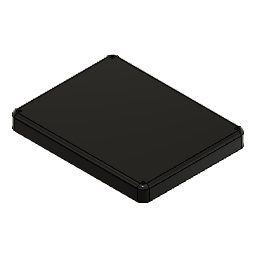
electronic_box (Autodesk Fusion 360 design; units mm, degrees)
Autodesk Fusion 360 part; units mm, degrees
note: some values were not read from the file. Set by a fixed rule: which sketch regions a step uses; which face or edge a step refers to.
sketch "Esquisse1" plane through (0, 0, 0) normal (0, 1, 0) x (1, 0, 0)
  line L0 (-100, 85) -> (100, 85)
  line L1 (110, 75) -> (110, -75)
  line L2 (100, -85) -> (-100, -85)
  line L3 (-110, -75) -> (-110, 75)
  line L4 (-110, 85) -> (110, -85) construction
  line L5 (110, 85) -> (-110, -85) construction
  arc A0 (-100, 85) -> (-110, 75) centre (-100, 75) ccw
  arc A1 (110, 75) -> (100, 85) centre (100, 75) ccw
  arc A2 (100, -85) -> (110, -75) centre (100, -75) ccw
  arc A3 (-110, -75) -> (-100, -85) centre (-100, -75) ccw
  arc A4 (-100, 82) -> (-107, 75) centre (-100, 75) ccw
  line L6 (-107, -75) -> (-107, 75)
  arc A5 (-107, -75) -> (-100, -82) centre (-100, -75) ccw
  line L7 (100, -82) -> (-100, -82)
  arc A6 (100, -82) -> (107, -75) centre (100, -75) ccw
  line L8 (107, 75) -> (107, -75)
  arc A7 (107, 75) -> (100, 82) centre (100, 75) ccw
  line L9 (-100, 82) -> (100, 82)
  dimension "d8" = 170
  dimension "d9" = 220
  dimension "d10" = 10
  dimension "d11" = 3
  constraint horizontal L0
  constraint perpendicular L0 L1
  constraint parallel L0 L2
  constraint parallel L1 L3
  constraint coincident L4 origin
  constraint coincident L5 origin
  constraint coincident L4.start L3
  constraint coincident L4.start L0
  constraint tangent L3 A0
  constraint tangent L0 A0
  constraint coincident L5.start L0
  constraint coincident L5.start L1
  constraint tangent L0 A1
  constraint tangent L1 A1
  constraint equal A0 A1
  constraint coincident L4.end L2
  constraint coincident L4.end L1
  constraint tangent L2 A2
  constraint tangent L1 A2
  constraint equal A0 A2
  constraint coincident L5.end L2
  constraint coincident L5.end L3
  constraint tangent L2 A3
  constraint tangent L3 A3
  constraint equal A0 A3
  measures "d8" distance of L4.start L5.end
  measures "d9" distance of L4.end L5.end
  measures "d10" radius of A0
extrude "Extrusion2" add sketch "Esquisse1" along normal blind 20 makes body 1
sketch "Esquisse2" plane through (0, 20, 0) normal (0, 1, 0) x (-1, 0, 0)
  arc A0 (107, 75) -> (100, 82) centre (100, 75) ccw
  line L0 (107, 75) -> (107, -75)
  arc A1 (100, -82) -> (107, -75) centre (100, -75) ccw
  line L1 (100, -82) -> (-100, -82)
  arc A2 (-107, -75) -> (-100, -82) centre (-100, -75) ccw
  line L2 (-107, -75) -> (-107, 75)
  arc A3 (-100, 82) -> (-107, 75) centre (-100, 75) ccw
  line L3 (-100, 82) -> (100, 82)
  arc A4 (100, -85) -> (110, -75) centre (100, -75) ccw
  line L4 (110, -75) -> (110, 75)
  arc A5 (110, 75) -> (100, 85) centre (100, 75) ccw
  line L5 (100, 85) -> (-100, 85)
  arc A6 (-100, 85) -> (-110, 75) centre (-100, 75) ccw
  line L6 (-110, 75) -> (-110, -75)
  arc A7 (-110, -75) -> (-100, -85) centre (-100, -75) ccw
  line L7 (-100, -85) -> (100, -85)
  line L8 (-110, 75) -> (-110, -75)
  arc A8 (-100, 85) -> (-110, 75) centre (-100, 75) ccw
  line L9 (100, 85) -> (-100, 85)
  circle A9 centre (100, 75) radius 0.001
  line L10 (110, -75) -> (110, 75)
  arc A10 (100, -85) -> (110, -75) centre (100, -75) ccw
  line L11 (-100, -85) -> (100, -85)
  circle A11 centre (-100, -75) radius 0.001
extrude "Extrusion3" add sketch "Esquisse2" along normal blind 3 contours A0 L0 A1 L1 A2 L2 A3 L3 | A4 L4 A5 L5 A6 L6 A7 L7 L8 A8 L9 L10 A10 L11 | A9 | A11 bodies 1
fillet "Congé1" radius 2 8 edges at (0, 20, -82) (104.9497, 20, -79.9497) (107, 20, 0) (104.9497, 20, 79.9497) (0, 20, 82) (-104.9497, 20, 79.9497) (-107, 20, 0) (-104.9497, 20, -79.9497) on bodies 1
fillet "Congé2" radius 5 8 edges at (0, 23, 85) (107.0711, 23, 82.0711) (110, 23, 0) (107.0711, 23, -82.0711) (0, 23, -85) (-107.0711, 23, -82.0711) (-110, 23, 0) (-107.0711, 23, 82.0711) on bodies 1
sketch "Esquisse3" plane through (0, 0, -85) normal (0, 0, -1) x (-1, 0, 0)
  line L0 (100, 18) -> (-100, 18)
  line L1 (-100, 18) -> (-100, 0)
  line L2 (-100, 0) -> (100, 0)
  line L3 (100, 0) -> (100, 18)
  line L4 (-58.4785, 6.134) -> (-73.4785, 6.134)
  line L5 (-73.4785, 6.134) -> (-73.4785, 13.134)
  line L6 (-73.4785, 13.134) -> (-58.4785, 13.134)
  line L7 (-58.4785, 13.134) -> (-58.4785, 6.134)
  line L8 (-39.7725, 5.6821) -> (-51.7725, 5.6821)
  line L9 (-51.7725, 5.6821) -> (-51.7725, 13.6821)
  line L10 (-51.7725, 13.6821) -> (-39.7725, 13.6821)
  line L11 (-39.7725, 13.6821) -> (-39.7725, 5.6821)
  circle A0 centre (-32.676, 9.0787) radius 2.5
  dimension "d20" = 15
  dimension "d21" = 7
  dimension "d24" = 12
  dimension "d25" = 8
  dimension "d26" = 5
  constraint horizontal L4
  constraint vertical L5
  constraint horizontal L6
  constraint vertical L7
  constraint horizontal L8
  constraint vertical L9
  constraint horizontal L10
  constraint vertical L11
  measures "d20" distance of L4.start L4.end
  measures "d21" distance of L4.start L6.end
  measures "d24" distance of L8.start L8.end
  measures "d25" distance of L8.start L10.end
  measures "d26" diameter of A0
extrude "Extrusion4" cut sketch "Esquisse3" against normal blind 30 contours L4 L5 L6 L7 | L8 L9 L10 L11 | A0 bodies 1
sketch "Esquisse4" plane through (0, 0, 0) normal (0, -1, 0) x (1, 0, 0)
  arc A0 (-100, 82) -> (-107, 75) centre (-100, 75) ccw
  line L0 (-100, 82) -> (100, 82)
  arc A1 (107, 75) -> (100, 82) centre (100, 75) ccw
  line L1 (107, 75) -> (107, -75)
  arc A2 (100, -82) -> (107, -75) centre (100, -75) ccw
  line L2 (100, -82) -> (-100, -82)
  arc A3 (-107, -75) -> (-100, -82) centre (-100, -75) ccw
  line L3 (-107, -75) -> (-107, 75)
  arc A4 (-110, -75) -> (-100, -85) centre (-100, -75) ccw
  line L4 (-100, -85) -> (100, -85)
  arc A5 (100, -85) -> (110, -75) centre (100, -75) ccw
  line L5 (110, -75) -> (110, 75)
  arc A6 (110, 75) -> (100, 85) centre (100, 75) ccw
  line L6 (100, 85) -> (-100, 85)
  arc A7 (-100, 85) -> (-110, 75) centre (-100, 75) ccw
  line L7 (-110, 75) -> (-110, -75)
sketch "Esquisse5" plane through (0, 20, 0) normal (0, -1, 0) x (1, 0, 0)
  line L0 (-100, -80) -> (100, -80)
  line L1 (105, -75) -> (105, 75)
  line L2 (100, 80) -> (-100, 80)
  line L3 (-105, 75) -> (-105, -75)
  circle A0 centre (-101, 76) radius 2
  circle A1 centre (-101, 76) radius 2
  circle A2 centre (-101, 76) radius 3
  line L4 (0, 100) -> (0, -84.8494) construction
  line L5 (-132.4366, 0.0945) -> (95, 0.0945) construction
  circle A3 centre (101, 76) radius 3
  circle A4 centre (101, 76) radius 2
  circle A5 centre (101, -75.811) radius 3
  circle A6 centre (101, -75.811) radius 2
  circle A7 centre (-101, -75.811) radius 3
  circle A8 centre (-101, -75.811) radius 2
  arc A9 (100, -80) -> (105, -75) centre (100, -75) ccw
  arc A10 (105, 75) -> (100, 80) centre (100, 75) ccw
  arc A11 (-100, 80) -> (-105, 75) centre (-100, 75) ccw
  arc A12 (-105, -75) -> (-100, -80) centre (-100, -75) ccw
  point P0 (-101, -75.811)
  dimension "d27" = 4
  dimension "d28" = 4
  dimension "d29" = 6
  dimension "d30" = 4
  dimension "d31" = 4
  dimension "d32" = 4
  dimension "d33" = 4
  constraint concentric A0 A2
  constraint perpendicular L2 L4
  constraint perpendicular L1 L5
  constraint symmetric A0 L4 A4
  constraint symmetric A2 L4 A3
  constraint symmetric A0 L5 A8
  constraint symmetric A0.centre L5 P0
  constraint symmetric A2 L5 A7
  constraint symmetric L5 A3 A5
  constraint symmetric L5 A4 A6
  measures "d27" diameter of A0
  measures "d28" diameter of A1
  measures "d29" diameter of A2
  measures "d30" distance of L2 A0.centre
  measures "d31" distance of L2 A0.centre
  measures "d32" distance of L3 A0.centre
  measures "d33" distance of L3 A0.centre
extrude "Extrusion5" add sketch "Esquisse5" along normal up to surface (20 mm away) contours A2 | A3 | A5 | A7 bodies 1
extrude "Extrusion6" cut sketch "Esquisse5" against normal blind 55 contours A0 A1 | A4 | A6 | A8 bodies 1
sketch "Esquisse6" plane through (0, 0, -85) normal (0, 0, -1) x (-1, 0, 0)
  line L0 (-73.4785, 6.134) -> (-73.4785, 13.134)
  line L1 (-73.4785, 13.134) -> (-58.4785, 13.134)
  line L2 (-58.4785, 13.134) -> (-58.4785, 6.134)
  line L3 (-58.4785, 6.134) -> (-73.4785, 6.134)
  line L4 (-51.7725, 5.6821) -> (-51.7725, 13.6821)
  line L5 (-51.7725, 13.6821) -> (-39.7725, 13.6821)
  line L6 (-39.7725, 13.6821) -> (-39.7725, 5.6821)
  line L7 (-39.7725, 5.6821) -> (-51.7725, 5.6821)
  circle A0 centre (-32.676, 9.0787) radius 2.5
  line L8 (100, 18) -> (-100, 18)
  line L9 (-100, 18) -> (-100, 0)
  line L10 (-100, 0) -> (100, 0)
  line L11 (100, 0) -> (100, 18)
  line L12 (95, 0) -> (10, 0)
  line L13 (10, 0) -> (10, 18)
  line L14 (10, 18) -> (95, 18)
  line L15 (95, 18) -> (95, 0)
  dimension "d39" = 85
  dimension "d45" = 5
  constraint horizontal L12
  constraint vertical L13
  constraint horizontal L14
  constraint vertical L15
  constraint coincident L8 L13.end
  constraint coincident L10 L12.start
  measures "d39" distance of L13 L15
  measures "d45" distance of L11 L15
extrude "Extrusion7" cut sketch "Esquisse6" against normal blind 25 contours L8 L10 L12 L13 L14 L15 bodies 1
sketch "Esquisse7" plane through (0, 0, 0) normal (0, -1, 0) x (1, 0, 0)
  line L0 (-95, -85) -> (-95, -82)
  line L1 (-95, -82) -> (-100, -82)
  arc A0 (-107, -75) -> (-100, -82) centre (-100, -75) ccw
  line L2 (-107, -75) -> (-107, 75)
  arc A1 (-100, 82) -> (-107, 75) centre (-100, 75) ccw
  line L3 (-100, 82) -> (100, 82)
  arc A2 (107, 75) -> (100, 82) centre (100, 75) ccw
  line L4 (107, 75) -> (107, -75)
  arc A3 (100, -82) -> (107, -75) centre (100, -75) ccw
  line L5 (100, -82) -> (-10, -82)
  line L6 (-10, -82) -> (-10, -85)
  line L7 (-10, -85) -> (100, -85)
  arc A4 (100, -85) -> (110, -75) centre (100, -75) ccw
  line L8 (110, -75) -> (110, 75)
  arc A5 (110, 75) -> (100, 85) centre (100, 75) ccw
  line L9 (100, 85) -> (-100, 85)
  arc A6 (-100, 85) -> (-110, 75) centre (-100, 75) ccw
  line L10 (-110, 75) -> (-110, -75)
  arc A7 (-110, -75) -> (-100, -85) centre (-100, -75) ccw
  line L11 (-100, -85) -> (-95, -85)
sketch "Esquisse8" plane through (0, 0, 0) normal (0, -1, 0) x (1, 0, 0)
  line L0 (-95, -82) -> (-95, -80)
  line L1 (-95, -80) -> (-90, -80)
  line L2 (-90, -80) -> (-90, -75)
  line L3 (-90, -75) -> (-98, -75)
  line L4 (-98, -75) -> (-98, -82)
  line L5 (-98, -82) -> (-95, -82)
  line L6 (-10, -82) -> (-10, -80)
  line L7 (-10, -80) -> (-15, -80)
  line L8 (-15, -80) -> (-15, -75)
  line L9 (-15, -75) -> (-5, -75)
  line L10 (-5, -75) -> (-5, -82)
  line L11 (-5, -82) -> (-10, -82)
  constraint vertical L0
  constraint perpendicular L0 L1
  constraint perpendicular L1 L2
  constraint perpendicular L2 L3
  constraint perpendicular L3 L4
  constraint perpendicular L0 L5
  constraint vertical L6
  constraint perpendicular L6 L7
  constraint perpendicular L7 L8
  constraint perpendicular L6 L9
  constraint perpendicular L9 L10
  constraint perpendicular L6 L11
extrude "Extrusion9" cut sketch "Esquisse8" against normal up to surface (20 mm away) bodies 1
extrude "Extrusion10" add sketch "Esquisse8" against normal up to surface (20 mm away) separate body makes body 2 at (-92.6667, 6.6667, -75) makes body 3 at (-11.6667, 13.3333, -75)
sketch "Esquisse9" plane through (0, 0, -80) normal (0, 0, -1) x (-1, 0, 0)
  line L0 (95, 20) -> (90, 20)
  line L1 (90, 20) -> (90, 0)
  line L2 (90, 0) -> (95, 0)
  line L3 (95, 0) -> (95, 20)
  line L4 (95, 5) -> (91, 5)
  line L5 (91, 5) -> (91, 9)
  line L6 (91, 9) -> (95, 9)
  line L7 (95, 9) -> (95, 5)
  line L8 (10, 5) -> (14, 5)
  line L9 (14, 5) -> (14, 9)
  line L10 (14, 9) -> (10, 9)
  line L11 (10, 9) -> (10, 5)
  constraint horizontal L4
  constraint vertical L5
  constraint horizontal L6
  constraint vertical L7
  constraint coincident L3 L4.start
  constraint horizontal L8
  constraint vertical L9
  constraint horizontal L10
  constraint vertical L11
extrude "Extrusion11" cut sketch "Esquisse9" against normal blind 4 contours L3 L4 L5 L6 L7 | L8 L9 L10 L11 bodies 2 3
